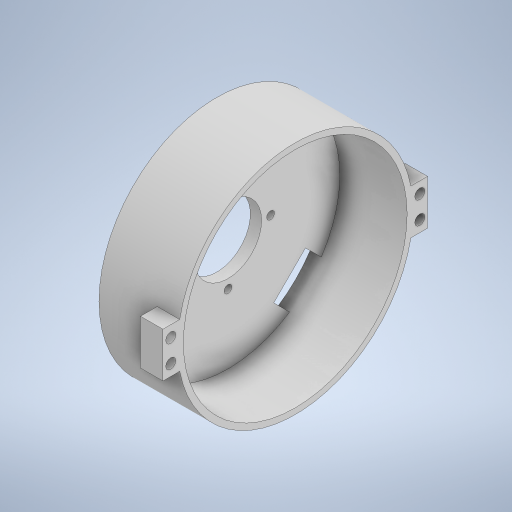
# Autodesk Inventor part: MotorHouse
Saved by Autodesk Inventor 2023 (Build 270158000, 158)
## iProperties
Created: 2023-02-23
Part Number: MotorHouse
Material: Generic
Document SubType Name: Sheet Metal
Designer: Charles Kelly
Density: 1 g/cm^3
Sheet Metal Rule: Default_mm
Appearance: Default
Author: Charles Kelly
Autodesk Inventor part; units mm, degrees
ref_plane "YZ Plane" through (0, 0, 0) normal (1, 0, 0) x (0, 1, 0)
ref_plane "XZ Plane" through (0, 0, 0) normal (0, 1, 0) x (-1, 0, 0)
ref_plane "XY Plane" through (0, 0, 0) normal (0, 0, 1) x (1, 0, 0)
sketch "Sketch1" plane through (0, 0, 0) normal (1, 0, 0) x (0, 1, 0)
  circle A0 centre (0, 0) radius 19
  circle A1 centre (0, -19) radius 1.75
  circle A2 centre (19, 0) radius 1.75
  circle A3 centre (0, 19) radius 1.75
  circle A4 centre (-19, 0) radius 1.75
  circle A5 centre (0, 0) radius 52.5
  circle A6 centre (0, 0) radius 40
  dimension "d0" = 38
  dimension "d1" = 3.5
  dimension "d4" = 360
  dimension "d6" = 105
  dimension "d7" = 80
  constraints: 6 centre point, 3 coincident, 1 vertical alignment, 11 other
  measures "d1" diameter of A1
  measures "d6" diameter of A5
  measures "d7" diameter of A6
extrude "Extrusion1" add sketch "Sketch1" along normal blind 5 contours A2 A0 A1 A4 A3 | A5 | A6
sketch "Sketch2" plane through (0, 0, 0) normal (-1, 0, 0) x (0, 0, 1)
  circle A0 centre (0, 0) radius 52.5
  circle A1 centre (0, 0) radius 49.875
  dimension "d10" = 105
  constraints: 2 centre point, 2 coincident
  measures "d10" diameter of A0
extrude "Extrusion2" add sketch "Sketch2" against normal blind 35
sketch "Sketch3" plane through (35, 0, 0) normal (1, 0, 0) x (0, 0, -1)
  circle A0 centre (0, 0) radius 52.5
  circle A1 centre (0, 0) radius 47.5 projected
  line L0 (-48.9952, 10) -> (-58.9952, 10)
  line L1 (-58.9952, 10) -> (-58.9952, -10)
  line L2 (-58.9952, -10) -> (-51.5388, -10)
  line L3 (-48.9952, 10) -> (-51.5388, 10)
  line L4 (-47.5, 0) -> (-55.5093, 0)
  line L5 (-55.5093, 0) -> (-55.5093, 5)
  circle A2 centre (-55.5093, 5) radius 2.25
  line L6 (-55.5093, 0) -> (-55.5093, -5)
  circle A3 centre (-55.5093, -5) radius 2.25
  line L7 (48.9952, -10) -> (58.9952, -10)
  line L8 (58.9952, -10) -> (58.9952, 10)
  line L9 (58.9952, 10) -> (51.5388, 10)
  line L10 (48.9952, -10) -> (51.5388, -10)
  line L11 (47.5, 0) -> (55.5093, 0)
  line L12 (55.5093, 0) -> (55.5093, -5)
  circle A4 centre (55.5093, -5) radius 2.25
  line L13 (55.5093, 0) -> (55.5093, 5)
  circle A5 centre (55.5093, 5) radius 2.25
  point P0 (51.5388, -10)
  point P1 (47.2562, -4.8066)
  point P2 (47.2562, 4.8066)
  point P3 (51.5388, -10)
  point P4 (-47.2562, 4.8066)
  point P5 (-47.2562, -4.8066)
  dimension "d14" = 10
  dimension "d15" = 20
  dimension "d17" = 5
  dimension "d18" = 4.5
  dimension "d19" = 5
  dimension "d20" = 4.5
  dimension "d23" = 360
  dimension "d33" = 105
  constraints: 28 end point, 5 centre point, 5 coincident, 4 point on line, 3 perpendicular, 2 point on circle, 1 horizontal, 1 horizontal alignment, 1 line through centre, 42 other
  measures "d14" distance of L0.start L0.end
  measures "d15" distance of L0.end L1.end
  measures "d17" distance of L4.end L5.end
  measures "d18" diameter of A2
  measures "d19" distance of L4.end L6.end
  measures "d20" diameter of A3
  measures "d33" diameter of A0
extrude "Extrusion3" add sketch "Sketch3" against normal blind 10 contours A0 L9 L8 L7 | A0 L2 L1 L0
sketch "Sketch4" plane through (5, 0, 0) normal (1, 0, 0) x (0, 0, -1)
  circle A0 centre (0, 0) radius 15
  line L0 (0, 0) -> (7.0711, 7.0711)
  line L1 (0, 0) -> (10, 0) construction
  line L2 (7.0711, 7.0711) -> (41.6219, -27.4797)
  circle A1 centre (0, 0) radius 49.875 projected
  line L3 (0, 0) -> (-7.0711, -7.0711)
  line L4 (-7.0711, -7.0711) -> (27.4797, -41.6219)
  line L5 (41.6219, -27.4797) -> (34.5508, -20.4087)
  line L6 (34.5508, -20.4087) -> (20.4087, -34.5508)
  point P0 (0.8346, -14.9768)
  point P1 (14.9768, -0.8346)
  point P2 (48.8622, 10)
  point P3 (-48.8622, 10)
  dimension "d27" = 30
  dimension "d28" = 10
  dimension "d29" = 45
  dimension "d30" = 10
  dimension "d34" = 10
  constraints: 14 end point, 3 perpendicular, 3 point on circle, 3 point on line, 1 centre point, 1 coincident, 1 equal length, 1 horizontal
  measures "d27" diameter of A0
  measures "d28" distance of L0.start L0.end
  measures "d29" angle of L1 L0
  measures "d30" distance of L3.start L3.end
  measures "d34" distance of L5.start L5.end
extrude "Extrusion4" cut sketch "Sketch4" against normal blind 10 contours A0 L2 L0 L3 L4 | L4 L3 L0 L2 A0 | L6 L2 A1 L4
equation "\"BendRadius\" = Thickness"
equation "\"BendReliefWidth\" = Thickness"
equation "\"BendReliefDepth\" = 0.5 * Thickness"
equation "\"CornerReliefSize\" = 4 * Thickness"
equation "\"MinimumRemnant\" = 2 * Thickness"
equation "\"TransitionRadius\" = BendRadius"
equation "\"JacobiRadiusSize\" = BendRadius"
equation "\"GapSize\" = Thickness"
equation "\"Thickness\" = 0.5"
body "Solid1"
